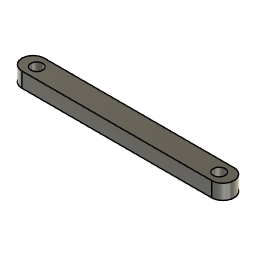
total_finger (Autodesk Fusion 360 archive; units mm, degrees)
design "fixador 1"
Autodesk Fusion 360 part; units mm, degrees
note: some values were not read from the file. Chosen so that the rebuilt part matches the saved one: which face or edge a step refers to. Set by a fixed rule: which sketch regions a step uses.
sketch "Esboço1" plane through (0, 0, 0) normal (0, 0, 1) x (1, 0, 0)
  line L0 (18.163, 18) -> (75.223, 18)
  line L1 (75.223, 18) -> (75.223, 12)
  line L2 (75.223, 12) -> (18.163, 12)
  line L3 (18.163, 12) -> (18.163, 18)
  circle A0 centre (22.163, 15) radius 1.6
  circle A1 centre (71.223, 15) radius 1.6
  dimension "d2" = 3.2
  dimension "d3" = 3.2
  dimension "d4" = 49.06
  dimension "d5" = 4
  dimension "d6" = 4
  dimension "d13" = 6
  dimension "d14" = 3
  constraint horizontal L0
  constraint vertical L1
  constraint horizontal L2
  constraint vertical L3
  measures "d2" diameter of A0
  measures "d3" diameter of A1
  measures "d4" distance of A0.centre A1.centre
  measures "d5" distance of L3 A0.centre
  measures "d6" distance of L1 A1.centre
  measures "d13" distance of L0.start L2.end
  measures "d14" distance of L0 A0.centre
extrude "Extrusão1" add sketch "Esboço1" along normal blind 4
fillet "Arredondamento3" radius 3 2 edges at (18.163, 18, 2) (18.163, 12, 2)
fillet "Arredondamento4" radius 3 2 edges at (75.223, 18, 2) (75.223, 12, 2)
scale "Escala1" factor 0.7 about (20.563, 15, 0) bodies 1
scale "Escala2" factor 1.14 about (20.983, 17.1, 2.8) bodies 1

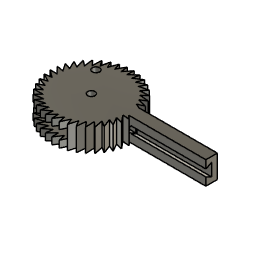
design "contato"
Autodesk Fusion 360 part; units mm, degrees
sketch "Esboço1" plane through (0, 0, 0) normal (0, 0, 1) x (1, 0, 0)
  circle A0 centre (0, 0) radius 15
  line L0 (5, 0) -> (30, 0)
  line L1 (30, 0) -> (30, 5)
  line L2 (30, 5) -> (5, 5)
  line L3 (5, 5) -> (5, 0)
  line L4 (-15, 0) -> (-18, 0)
  line L5 (-18, 0) -> (-14.8037, -2.4188)
  dimension "d1" = 30
  dimension "d41" = 3
  constraint coincident A0.centre origin
  constraint horizontal L0
  constraint vertical L1
  constraint horizontal L2
  constraint vertical L3
  constraint coincident A0 L4.start
  constraint horizontal L4
  constraint coincident A0 L5.end
  measures "d1" diameter of A0
  measures "d41" distance of L4.start L4.end
extrude "Extrusão1" add sketch "Esboço1" along normal blind 10 makes body 1
extrude "Extrusão2" add sketch "Esboço1" along normal blind 10 contours A0 L4 L5 bodies 1
pattern_circular "Padrão circular1" count 39 over 360 about axis through (0, 0, 10) along (0, 0, 1) of "Extrusão2"
sketch "Esboço2" plane through (30, 0, 0) normal (1, 0, 0) x (0, 1, 0)
  line L0 (0, 0) -> (5, 0)
  line L1 (5, 0) -> (5, 10)
  line L2 (5, 10) -> (0, 10)
  line L3 (0, 10) -> (0, 0)
  line L4 (0, 6.2) -> (2.0156, 7.2)
  line L5 (2.0156, 7.2) -> (2.0156, 2.8)
  line L6 (2.0156, 2.8) -> (0, 3.8)
  line L7 (0, 6.2) -> (0, 3.8)
  dimension "d8" = 4.4
  dimension "d9" = 2.25
  dimension "d10" = 2.25
  dimension "d11" = 2.4
  dimension "d12" = 3.8
  constraint coincident L3 L4.start
  constraint parallel L3 L5
  constraint coincident L3 L6.end
  measures "d8" distance of L4.end L5.end
  measures "d9" distance of L4.start L4.end
  measures "d10" distance of L5.end L6.end
  measures "d11" distance of L4.start L6.end
  measures "d12" distance of L2.end L4.start
extrude "Extrusão3" cut sketch "Esboço2" against normal blind 19 contours L3 L4 L5 L6 L7 bodies 1
sketch "Esboço3" plane through (0, 0, 10) normal (0, 0, 1) x (-1, 0, 0)
  line L0 (18, 0) -> (14.8178, 2.4081)
  line L1 (15.0122, 0) -> (18, 0)
  line L2 (17.7669, 2.8874) -> (14.2396, 4.7539)
  line L3 (14.8178, 2.4081) -> (17.7669, 2.8874)
  line L4 (17.0737, 5.7) -> (13.2927, 6.9765)
  line L5 (14.2396, 4.7539) -> (17.0737, 5.7)
  line L6 (15.9382, 8.365) -> (12.0014, 9.0185)
  line L7 (13.2927, 6.9765) -> (15.9382, 8.365)
  line L8 (14.39, 10.8134) -> (10.3993, 10.8268)
  line L9 (12.0014, 9.0185) -> (14.39, 10.8134)
  line L10 (12.469, 12.9816) -> (8.5279, 12.3548)
  line L11 (10.3993, 10.8268) -> (12.469, 12.9816)
  line L12 (10.2252, 14.8137) -> (6.4356, 13.5628)
  line L13 (8.5279, 12.3548) -> (10.2252, 14.8137)
  line L14 (7.7165, 16.2621) -> (4.1767, 14.4195)
  line L15 (6.4356, 13.5628) -> (7.7165, 16.2621)
  line L16 (5.0079, 17.2893) -> (1.8095, 14.9028)
  line L17 (4.1767, 14.4195) -> (5.0079, 17.2893)
  line L18 (2.1697, 17.8688) -> (-0.6045, 15)
  line L19 (1.8095, 14.9028) -> (2.1697, 17.8688)
  line L20 (-0.7248, 17.9854) -> (-3.0028, 14.7088)
  line L21 (-0.6045, 15) -> (-0.7248, 17.9854)
  line L22 (-3.6005, 17.6362) -> (-5.3234, 14.0367)
  line L23 (-3.0028, 14.7088) -> (-3.6005, 17.6362)
  line L24 (-5.3234, 14.0367) -> (-6.3829, 16.8303)
  line L25 (-9, 15.5885) -> (-9.4944, 11.6285)
  line L26 (-11.384, 13.9429) -> (-11.2368, 9.9549)
  line L27 (-9.4944, 11.6285) -> (-11.384, 13.9429)
  line L28 (-13.4732, 11.9362) -> (-12.6882, 8.0235)
  line L29 (-11.2368, 9.9549) -> (-13.4732, 11.9362)
  line L30 (-15.2134, 9.6204) -> (-13.8109, 5.8843)
  line L31 (-12.6882, 8.0235) -> (-15.2134, 9.6204)
  line L32 (-16.5596, 7.0554) -> (-14.576, 3.5927)
  line L33 (-13.8109, 5.8843) -> (-16.5596, 7.0554)
  line L34 (-14.576, 3.5927) -> (-17.477, 4.3077)
  line L35 (-15.8671, -5) -> (-13.8109, -5.8843)
  line L36 (-16.5596, -7.0554) -> (-12.6882, -8.0235)
  line L37 (-13.8109, -5.8843) -> (-16.5596, -7.0554)
  line L38 (-15.2134, -9.6204) -> (-11.2368, -9.9549)
  line L39 (-12.6882, -8.0235) -> (-15.2134, -9.6204)
  line L40 (-30, 0) -> (-30, -5)
  line L41 (-30, -5) -> (-15.8671, -5)
  circle A0 centre (0, 0) radius 1.6
  line L42 (-11.2368, -9.9549) -> (-13.4732, -11.9362)
  line L43 (-13.4732, -11.9362) -> (-9.4944, -11.6285)
  line L44 (-9.4944, -11.6285) -> (-11.384, -13.9429)
  line L45 (-11.384, -13.9429) -> (-7.5061, -13.001)
  line L46 (-7.5061, -13.001) -> (-9, -15.5885)
  line L47 (-9, -15.5885) -> (-5.3234, -14.0367)
  line L48 (-5.3234, -14.0367) -> (-6.3829, -16.8303)
  line L49 (-6.3829, -16.8303) -> (-3.0028, -14.7088)
  line L50 (-3.0028, -14.7088) -> (-3.6005, -17.6362)
  line L51 (-3.6005, -17.6362) -> (-0.6045, -15)
  line L52 (-0.6045, -15) -> (-0.7248, -17.9854)
  line L53 (-0.7248, -17.9854) -> (1.8095, -14.9028)
  line L54 (1.8095, -14.9028) -> (2.1697, -17.8688)
  line L55 (2.1697, -17.8688) -> (4.1767, -14.4195)
  line L56 (4.1767, -14.4195) -> (5.0079, -17.2893)
  line L57 (5.0079, -17.2893) -> (6.4356, -13.5628)
  line L58 (6.4356, -13.5628) -> (7.7165, -16.2621)
  line L59 (7.7165, -16.2621) -> (8.5279, -12.3548)
  line L60 (8.5279, -12.3548) -> (10.2252, -14.8137)
  line L61 (10.2252, -14.8137) -> (10.3993, -10.8268)
  line L62 (10.3993, -10.8268) -> (12.469, -12.9816)
  line L63 (12.469, -12.9816) -> (12.0014, -9.0185)
  line L64 (12.0014, -9.0185) -> (14.39, -10.8134)
  line L65 (14.39, -10.8134) -> (13.2927, -6.9765)
  line L66 (-6.3829, 16.8303) -> (-7.5061, 13.001)
  line L67 (-7.5061, 13.001) -> (-9, 15.5885)
  line L68 (-17.477, 4.3077) -> (-14.9635, 1.208)
  line L69 (-14.9635, 1.208) -> (-17.9416, 1.4484)
  line L70 (-17.9416, 1.4484) -> (-16.3178, 0)
  line L71 (-16.3178, 0) -> (-30, 0)
  line L72 (13.2927, -6.9765) -> (15.9382, -8.365)
  line L73 (15.9382, -8.365) -> (14.2396, -4.7539)
  line L74 (14.2396, -4.7539) -> (17.0737, -5.7)
  line L75 (17.0737, -5.7) -> (14.8178, -2.4081)
  line L76 (14.8178, -2.4081) -> (17.7669, -2.8874)
  line L77 (17.7669, -2.8874) -> (15.0122, 0)
  dimension "d15" = 3.2
  constraint coincident A0.centre origin
  measures "d15" diameter of A0
extrude "Extrusão4" cut sketch "Esboço3" against normal blind 10 contours A0 bodies 1
ref_plane "Plano de trabalho1" through (0, 0, 12.125) normal (0, -1, 0) x (0, 0, 1)
ref_plane "Plano de trabalho2" through (0, 25, 12.125) normal (0, -1, 0) x (0, 0, 1)
sketch "Esboço4" plane through (0, 25, 0) normal (0, -1, 0) x (0, 0, 1)
  line L0 (3, -5) -> (7, -5)
  line L1 (7, -5) -> (7, 21.5806)
  line L2 (7, 21.5806) -> (3, 21.5806)
  line L3 (3, 21.5806) -> (3, -5)
  dimension "d20" = 4
  dimension "d21" = 3
  constraint horizontal L0
  constraint vertical L1
  constraint horizontal L2
  constraint vertical L3
  measures "d20" distance of L0.start L0.end
  measures "d21" distance of origin L3
extrude "Extrusão5" cut sketch "Esboço4" along normal blind 45 bodies 1
sketch "Esboço5" plane through (0, 0, 3) normal (0, 0, 1) x (-1, 0, 0)
  line L0 (10.2252, 14.8137) -> (6.4356, 13.5628)
  line L1 (-5, 14.7123) -> (-5, -15.9623)
  circle A0 centre (8, -10) radius 1.6
  line L2 (6.4356, 13.5628) -> (7.7165, 16.2621)
  circle A1 centre (0, 0) radius 1.6
  line L3 (15.0122, 0) -> (18, 0)
  line L4 (18, 0) -> (14.8178, 2.4081)
  line L5 (14.8178, 2.4081) -> (17.7669, 2.8874)
  line L6 (17.7669, 2.8874) -> (14.2396, 4.7539)
  line L7 (14.2396, 4.7539) -> (17.0737, 5.7)
  line L8 (17.0737, 5.7) -> (13.2927, 6.9765)
  line L9 (13.2927, 6.9765) -> (15.9382, 8.365)
  line L10 (15.9382, 8.365) -> (12.0014, 9.0185)
  line L11 (12.0014, 9.0185) -> (14.39, 10.8134)
  line L12 (14.39, 10.8134) -> (10.3993, 10.8268)
  line L13 (10.3993, 10.8268) -> (12.469, 12.9816)
  line L14 (12.469, 12.9816) -> (8.5279, 12.3548)
  line L15 (8.5279, 12.3548) -> (10.2252, 14.8137)
  line L16 (7.7165, 16.2621) -> (4.1767, 14.4195)
  line L17 (-5, -15.9623) -> (-3.0028, -14.7088)
  line L18 (-3.0028, -14.7088) -> (-3.6005, -17.6362)
  line L19 (-3.6005, -17.6362) -> (-0.6045, -15)
  line L20 (-0.6045, -15) -> (-0.7248, -17.9854)
  line L21 (-0.7248, -17.9854) -> (1.8095, -14.9028)
  line L22 (1.8095, -14.9028) -> (2.1697, -17.8688)
  line L23 (2.1697, -17.8688) -> (4.1767, -14.4195)
  line L24 (4.1767, -14.4195) -> (5.0079, -17.2893)
  line L25 (5.0079, -17.2893) -> (6.4356, -13.5628)
  line L26 (6.4356, -13.5628) -> (7.7165, -16.2621)
  line L27 (7.7165, -16.2621) -> (8.5279, -12.3548)
  line L28 (8.5279, -12.3548) -> (10.2252, -14.8137)
  line L29 (10.2252, -14.8137) -> (10.3993, -10.8268)
  line L30 (10.3993, -10.8268) -> (12.469, -12.9816)
  line L31 (12.469, -12.9816) -> (12.0014, -9.0185)
  line L32 (12.0014, -9.0185) -> (14.39, -10.8134)
  line L33 (14.39, -10.8134) -> (13.2927, -6.9765)
  line L34 (4.1767, 14.4195) -> (5.0079, 17.2893)
  line L35 (5.0079, 17.2893) -> (1.8095, 14.9028)
  line L36 (1.8095, 14.9028) -> (2.1697, 17.8688)
  line L37 (2.1697, 17.8688) -> (-0.6045, 15)
  line L38 (-0.6045, 15) -> (-0.7248, 17.9854)
  line L39 (-0.7248, 17.9854) -> (-3.0028, 14.7088)
  line L40 (13.2927, -6.9765) -> (15.9382, -8.365)
  line L41 (15.9382, -8.365) -> (14.2396, -4.7539)
  line L42 (14.2396, -4.7539) -> (17.0737, -5.7)
  line L43 (17.0737, -5.7) -> (14.8178, -2.4081)
  line L44 (14.8178, -2.4081) -> (17.7669, -2.8874)
  line L45 (17.7669, -2.8874) -> (15.0122, 0)
  line L46 (-3.0028, 14.7088) -> (-3.6005, 17.6362)
  line L47 (-3.6005, 17.6362) -> (-5, 14.7123)
  point P0 (0, 0)
  point P1 (0, 0)
  point P2 (0, 0)
  point P3 (0, 0)
  point P4 (0, 0)
  point P5 (0, 0)
  point P6 (0, 0)
  point P7 (0, 0)
  point P8 (0, 0)
  point P9 (0, 0)
  point P10 (0, 0)
  point P11 (0, 0)
  point P12 (0, 0)
  point P13 (0, 0)
  point P14 (0, 0)
  point P15 (0, 0)
  point P16 (0, 0)
  point P17 (0, 0)
  point P18 (0, 0)
  point P19 (0, 0)
  point P20 (0, 0)
  point P21 (0, 0)
  point P22 (0, 0)
  point P23 (0, 0)
  point P24 (0, 0)
  point P25 (0, 0)
  point P26 (0, 0)
  point P27 (0, 0)
  point P28 (0, 0)
  point P29 (0, 0)
  point P30 (0, 0)
  point P31 (0, 0)
  point P32 (0, 0)
  point P33 (0, 0)
  point P34 (0, 0)
  point P35 (0, 0)
  point P36 (0, 0)
  point P37 (0, 0)
  point P38 (0, 0)
  point P39 (0, 0)
  point P40 (0, 0)
  point P41 (0, 0)
  point P42 (0, 0)
  point P43 (0, 0)
  point P44 (0, 0)
  point P45 (0, 0)
  point P46 (0, 0)
  point P47 (0, 0)
  point P48 (0, 0)
  point P49 (0, 0)
  point P50 (0, 0)
  point P51 (0, 0)
  point P52 (0, 0)
  point P53 (0, 0)
  point P54 (0, 0)
  point P55 (0, 0)
  point P56 (0, 0)
  point P57 (0, 0)
  point P58 (0, 0)
  point P59 (0, 0)
  point P60 (0, 0)
  point P61 (0, 0)
  dimension "d24" = 3.2
  measures "d24" diameter of A0
extrude "Extrusão6" cut sketch "Esboço5" against normal blind 6 contours A0 bodies 1
extrude "Extrusão7" cut sketch "Esboço5" along normal blind 7 contours A0 bodies 1
copy_body "Corpo -> Componente1" bodies 1 removing the originals makes body 2 in component "Component"
sketch "Esboço6" plane through (30, 0, 0) normal (1, 0, 0) x (0, 1, 0)
  line L0 (0, 6.2) -> (2.0156, 7.2)
  line L1 (2.0156, 7.2) -> (2.0156, 2.8)
  line L2 (2.0156, 2.8) -> (0, 3.8)
  line L3 (0, 3.8) -> (0, 0)
  line L4 (0, 0) -> (5, 0)
  line L5 (5, 0) -> (5, 10)
  line L6 (5, 10) -> (0, 10)
  line L7 (0.2342, 6.2703) -> (2.2498, 7.2703)
  line L8 (2.2498, 7.2703) -> (2.2498, 2.8703)
  line L9 (2.2498, 2.8703) -> (0, 2.8407)
  line L10 (0.2342, 6.2703) -> (0, 2.8407)
  line L11 (0, 10) -> (0, 6.2)
  dimension "d31" = 2.25
  dimension "d32" = 4.4
  dimension "d33" = 2.25
  dimension "d34" = 0.2445
  constraint parallel L0 L7
  constraint coincident L3 L9.end
  measures "d31" distance of L7.start L7.end
  measures "d32" distance of L7.end L8.end
  measures "d33" distance of L8.end L9.end
  measures "d34" distance of L0.start L7.start
extrude "Extrusão2'" add 1 faces at (11, 1.3437, 5.4) along direction (1, 0, 0) blind 3.66 on bodies 2 bodies 2 in component "Component"
extrude "Extrusão3'" add 1 faces at (30, 4.0052, 4.2667) along direction (1, 0, 0) blind 20 on bodies 2 bodies 2 in component "Component"
scale "Escala3" factor 0.7 about (16.3178, 0, 6.2) bodies 2 in component "Component"
scale "Escala4" factor 1.14 about (16.3178, 0, 6.2) bodies 2 in component "Component"
sketch "Esboço7" plane through (43.1962, 0, 0) normal (1, 0, 0) x (0, 1, 0)
  line L0 (0, 6.2) -> (1.6084, 6.998)
  line L1 (1.6084, 6.998) -> (1.6084, 3.4868)
  line L2 (1.6084, 3.4868) -> (0, 4.2848)
  line L3 (0, 4.2848) -> (0, 1.2524)
  line L4 (0, 1.2524) -> (3.99, 1.2524)
  line L5 (3.99, 1.2524) -> (3.99, 9.2324)
  line L6 (3.99, 9.2324) -> (0, 9.2324)
  line L7 (0, 9.2324) -> (0, 6.2)
  line L8 (0, 6.4424) -> (2.0156, 7.4424)
  line L9 (2.0156, 7.4424) -> (2.0156, 3.0424)
  line L10 (2.0156, 3.0424) -> (0, 4.0424)
  line L11 (0, 6.4424) -> (0, 4.0424)
  dimension "d44" = 2.25
  dimension "d45" = 4.4
  dimension "d46" = 2.25
  dimension "d47" = 2.79
  constraint parallel L0 L8
  constraint vertical L9
  constraint coincident L3 L10.end
  constraint parallel L3 L11
  measures "d44" distance of L8.start L8.end
  measures "d45" distance of L8.end L9.end
  measures "d46" distance of L9.end L10.end
  measures "d47" distance of L6.end L8.start
extrude "Extrusão4'" cut sketch "Esboço7" against normal blind 26 contours L0 L1 L2 L3 L7 L8 L9 L10 L11 bodies 2 in component "Component"
component "Component" placed x (1, 0, 0) y (0, 1, 0) z (0, 0, 1) at (0, 0, 0)

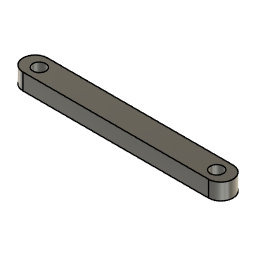
design "fixador 2"
Autodesk Fusion 360 part; units mm, degrees
sketch "Esboço1" plane through (0, 0, 0) normal (0, 0, 1) x (1, 0, 0)
  line L0 (16.7794, 7) -> (68.3114, 7)
  line L1 (68.3114, 7) -> (68.3114, 13)
  line L2 (68.3114, 13) -> (16.7794, 13)
  line L3 (16.7794, 13) -> (16.7794, 7)
  circle A0 centre (20.7794, 10) radius 1.6
  circle A1 centre (64.3114, 10) radius 1.6
  dimension "d1" = 3.2
  dimension "d2" = 3.2
  dimension "d3" = 43.532
  dimension "d4" = 4
  dimension "d6" = 6
  dimension "d7" = 3
  dimension "d14" = 4
  constraint horizontal L0
  constraint vertical L1
  constraint horizontal L2
  constraint vertical L3
  measures "d1" diameter of A0
  measures "d2" diameter of A1
  measures "d3" distance of A0.centre A1.centre
  measures "d4" distance of L3 A0.centre
  measures "d6" distance of L0.start L2.end
  measures "d7" distance of L0 A0.centre
  measures "d14" distance of L1 A1.centre
extrude "Extrusão1" add sketch "Esboço1" along normal blind 4 makes body 1
fillet "Arredondamento1" radius 3 2 edges at (16.7794, 13, 2) (16.7794, 7, 2) on bodies 1
fillet "Arredondamento2" radius 3 2 edges at (68.3114, 13, 2) (68.3114, 7, 2) on bodies 1
copy_body "Corpo -> Componente1" bodies 1 removing the originals makes body 2 in component "Component"
scale "Escala1" factor 0.7 about (65.3114, 13, 4) bodies 2 in component "Component"
scale "Escala2" factor 1.14 about (33.439, 8.8, 1.2) bodies 2 in component "Component"
component "Component" placed x (1, 0, 0) y (0, 1, 0) z (0, 0, 1) at (0, 0, 0)

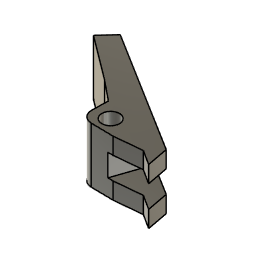
design "chave"
Autodesk Fusion 360 part; units mm, degrees
sketch "Esboço1" plane through (0, 0, 0) normal (0, 0, 1) x (1, 0, 0)
  line L0 (71.5982, 50.9917) -> (71.5183, 46.0145)
  line L1 (71.5982, 50.9917) -> (65.5982, 51.0881)
  line L2 (65.5989, 51.131) -> (65.5183, 46.1108)
  line L3 (65.5183, 46.1108) -> (71.5183, 46.0145)
  line L4 (64.2741, 55.8922) -> (67.524, 51.0571)
  circle A0 centre (68.5577, 48.5402) radius 1.6
  line L5 (76.5, 46.5) -> (79.1605, 44.7883)
  line L6 (79.1605, 44.7883) -> (78.4098, 48.7074)
  line L7 (64.2741, 55.8922) -> (62, 54)
  line L8 (62, 54) -> (65.5982, 51.0881)
  line L9 (64.2741, 55.8922) -> (71.5982, 50.9917)
  line L10 (71.5183, 46.0145) -> (76.5, 46.5)
  line L11 (78.4098, 48.7074) -> (71.5982, 50.9917)
  line L12 (62, 54) -> (54, 60)
  line L13 (54, 60) -> (56.3195, 62.5072)
  line L14 (56.3195, 62.5072) -> (64.2741, 55.8922)
  line L15 (56.3195, 62.5072) -> (78.4098, 48.7074)
  dimension "d1" = 3.2
  dimension "d12" = 46.4
  dimension "d14" = 2.5
  dimension "d15" = 6
  dimension "d16" = 3
  constraint perpendicular L0 L1
  constraint perpendicular L1 L2
  constraint perpendicular L0 L3
  constraint coincident L1 L4.end
  measures "d1" diameter of A0
  measures "d12" angle of L5 L6
  measures "d14" distance of L1 A0.centre
  measures "d15" horizontal distance of L0.end L2.end
  measures "d16" distance of L2 A0.centre
extrude "Extrusão1" add sketch "Esboço1" along normal blind 10 contours L0 L5 L6 L10 L11 | L0 L1 L2 L3 | L1 L4 L9 | L1 L4 L7 L8 | L7 L12 L13 L14
fillet "Arredondamento1" radius 2 1 edges at (65.5183, 46.1108, 5)
sketch "Esboço3" plane through (22.9508, 67.526, 0) normal (0.321801, 0.946807, 0) x (-0.946807, 0.321801, 0)
  line L0 (-58.5145, 0) -> (-51.3806, 0)
  line L1 (-51.3806, 10) -> (-58.5145, 10)
  line L2 (-58.5145, 10) -> (-58.5145, 0)
  line L3 (-62.3427, 3) -> (-52, 3)
  line L4 (-52, 3) -> (-52, 7)
  line L5 (-52, 7) -> (-62.3427, 7)
  line L6 (-62.3427, 7) -> (-62.3427, 3)
  line L7 (-51.3806, 0) -> (-51.3806, 10)
  dimension "d29" = 4
  dimension "d30" = 3
  constraint horizontal L3
  constraint vertical L4
  constraint horizontal L5
  constraint vertical L6
  measures "d29" distance of L3.end L4.end
  measures "d30" distance of L0 L3
extrude "Extrusão3" cut sketch "Esboço3" against normal blind 8 contours L2 L3 L5 L6 | L2 L3 L4 L5
sketch "Esboço4" plane through (0.7573, 47.151, 0) normal (-0.016059, -0.999871, 0) x (0.999871, -0.016059, 0)
  line L0 (69.8177, 7) -> (70.7701, 7)
  line L1 (70.7701, 10) -> (66.7694, 10)
  line L2 (66.7694, 10) -> (66.7694, 0)
  line L3 (66.7694, 0) -> (70.7701, 0)
  line L4 (70.7701, 3) -> (69.8177, 3)
  line L5 (69.8177, 3) -> (69.8177, 7)
  circle A0 centre (68, 5) radius 1
  line L6 (70.7701, 7) -> (70.7701, 10)
  line L7 (70.7701, 0) -> (70.7701, 3)
scale "Escala1" factor 0.7 about (72.1847, 50.7924, 3) bodies 1
scale "Escala2" factor 1.14 about (68.5258, 49.2158, 0.9) bodies 1
extrude "Extrusão6" cut 1 faces at (76.0121, 49.8863, 4.358) along direction (0.321801, 0.946807, 0) blind 7
sketch "Esboço6" plane through (0, 0, 8.88) normal (0, 0, 1) x (-1, 0, 0)
  arc A0 (-67.4028, -48.873) -> (-68.973, -47.2516) centre (-68.9986, -48.8474) ccw
  line L0 (-68.973, -47.2516) -> (-72.1652, -47.2003)
  line L1 (-72.1652, -47.2003) -> (-76.1406, -47.5878)
  line L2 (-76.1406, -47.5878) -> (-78.2636, -46.2219)
  line L3 (-78.2636, -46.2219) -> (-77.6646, -49.3492)
  line L4 (-77.6646, -49.3492) -> (-72.229, -51.1721)
  line L5 (-72.229, -51.1721) -> (-66.3843, -55.0827)
  line L6 (-66.3843, -55.0827) -> (-60.0366, -60.3615)
  line L7 (-60.0366, -60.3615) -> (-58.1856, -58.3608)
  line L8 (-58.1856, -58.3608) -> (-64.5696, -53.5728)
  line L9 (-64.5696, -53.5728) -> (-67.441, -51.249)
  line L10 (-67.441, -51.249) -> (-67.4028, -48.873)
  circle A1 centre (-69.8026, -49.2158) radius 1.2768
  line L11 (-60.0366, -60.3615) -> (-77.6646, -49.3492)
  constraint coincident L6.end L7.start
  constraint coincident L3.end L4.start
extrude "Extrusão7" add sketch "Esboço6" against normal blind 8 contours L4 L5 L6 L11
extrude "Extrusão8" cut 1 faces at (76.0089, 49.9045, 4.358) along direction (0.31796, 0.948104, 0) blind 4.5
sketch "Esboço7" plane through (0.7765, 48.3469, 0) normal (-0.016059, -0.999871, 0) x (0.999871, -0.016059, 0)
  line L0 (71.3979, 3.294) -> (70.6379, 3.294)
  line L1 (70.6379, 3.294) -> (70.6379, 6.486)
  line L2 (70.6379, 6.486) -> (71.3979, 6.486)
  line L3 (71.3979, 6.486) -> (71.3979, 8.88)
  line L4 (71.3979, 8.88) -> (68.2053, 8.88)
  line L5 (68.2053, 8.88) -> (68.2053, 0.9)
  line L6 (68.2053, 0.9) -> (71.3979, 0.9)
  line L7 (71.3979, 0.9) -> (71.3979, 3.294)
  line L8 (68.7249, 6.435) -> (70, 6.435)
  line L9 (70, 6.435) -> (70, 3.435)
  line L10 (70, 3.435) -> (68.7249, 3.435)
  line L11 (68.7249, 3.435) -> (68.7249, 6.435)
  dimension "d47" = 3
  constraint horizontal L8
  constraint vertical L9
  constraint horizontal L10
  constraint vertical L11
  measures "d47" distance of L8.start L10.end
extrude "Extrusão9" add sketch "Esboço7" along normal blind 2 contours L8 L9 L10 L11
sketch "Esboço8" plane through (69.991, -1.1241, 0) normal (0.999871, -0.016059, 0) x (0.016059, 0.999871, 0)
  line L0 (48.3531, 3.435) -> (48.3531, 6.435)
  line L1 (48.3531, 6.435) -> (46.3531, 6.435)
  line L2 (46.3531, 6.435) -> (46.3531, 3.435)
  line L3 (46.3531, 3.435) -> (48.3531, 3.435)
  line L4 (46.3531, 6.435) -> (47.3531, 6.435)
  line L5 (47.3531, 6.435) -> (47.3531, 3.435)
  line L6 (47.3531, 3.435) -> (46.3531, 3.435)
  line L7 (46.3531, 3.435) -> (46.3531, 6.435)
  constraint horizontal L4
  constraint vertical L5
  constraint horizontal L6
  constraint vertical L7
  constraint midpoint L3 L5.end
  constraint coincident L1.end L2.start
sketch "Esboço9" plane through (0, 0, 6.435) normal (0, 0, 1) x (-1, 0, 0)
  line L0 (-70.7675, -47.2228) -> (-69.4925, -47.2432)
  line L1 (-69.4925, -47.2432) -> (-69.4604, -45.2435)
  line L2 (-69.4604, -45.2435) -> (-70.7354, -45.223)
  line L3 (-70.7354, -45.223) -> (-70.7675, -47.2228)
  line L4 (-71.4473, -45.2116) -> (-72.2432, -45.6989)
  dimension "d52" = -3.3
  constraint coincident L2 L4.start
extrude "Extrusão11" cut sketch "Esboço9" against normal blind 3.3
